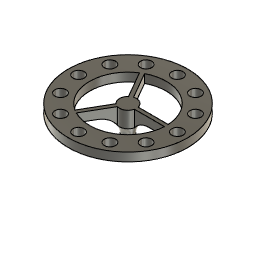
Wheel (Autodesk Fusion 360 design; units mm, degrees)
Autodesk Fusion 360 part; units mm, degrees
sketch "스케치1" plane through (0, 0, 0) normal (0, 0, 1) x (1, 0, 0)
  circle A0 centre (0, 0) radius 1.25
  circle A1 centre (0, 0) radius 3.3
  dimension "d1" = 2.5
  dimension "d2" = 6.6
  constraint coincident A0.centre A1.centre
  measures "d1" diameter of A0
  measures "d2" diameter of A1
extrude "돌출1" add sketch "스케치1" along normal blind 20
sketch "스케치2" plane through (0, 0, 20) normal (0, 0, 1) x (-1, 0, 0)
  circle A0 centre (0, 0) radius 35
  circle A1 centre (0, 0) radius 22.5
  circle A2 centre (0, 0) radius 3.3
  line L0 (-3.0194, -1.0904) -> (-22.4736, -1.0904)
  line L1 (-3.0232, 1.0832) -> (-22.4739, 1.0832)
  circle A3 centre (0, 0) radius 5
  line L2 (2.454, -2.0697) -> (12.1811, -18.9175)
  line L3 (0.5736, -3.1598) -> (10.2989, -20.0046)
  line L4 (0.5654, 3.16) -> (10.2925, 20.0079)
  line L5 (2.4497, 2.0766) -> (12.175, 18.9214)
  dimension "d5" = 70
  dimension "d11" = 45
  dimension "d21" = 10
  dimension "d32" = 360
  constraint coincident A0.centre A1.centre
  constraint concentric A1 A3
  constraint coincident A1 L1.end
  constraint horizontal L1
  constraint coincident A1 L0.end
  constraint horizontal L0
  measures "d5" diameter of A0
  measures "d11" diameter of A1
  measures "d21" diameter of A3
extrude "돌출3" add sketch "스케치2" along normal blind 5 contours A0 | A1 A3 L4 L5 | A1 A3 L2 L3 | A2 A3 L4 L5 | A2 A3 L2 L5 | A2 A3 L2 L3 | A1 L0 L1 A3 | A2 L1 A3 L4 | A2 | A2 L0 A3 L3 | A2 L0 L1 A3
sketch "스케치3" plane through (0, 0, 25) normal (0, 0, 1) x (-1, 0, 0)
  circle A0 centre (-29, 0) radius 3.3
  circle A1 centre (-25.1147, -14.5) radius 3.3
  circle A2 centre (-14.5, -25.1147) radius 3.3
  circle A3 centre (0, -29) radius 3.3
  circle A4 centre (14.5, -25.1147) radius 3.3
  circle A5 centre (25.1147, -14.5) radius 3.3
  circle A6 centre (29, 0) radius 3.3
  circle A7 centre (25.1147, 14.5) radius 3.3
  circle A8 centre (14.5, 25.1147) radius 3.3
  circle A9 centre (0, 29) radius 3.3
  circle A10 centre (-14.5, 25.1147) radius 3.3
  circle A11 centre (-25.1147, 14.5) radius 3.3
  dimension "d33" = 6.6
  dimension "d40" = 360
  measures "d33" diameter of A0
extrude "돌출7" cut sketch "스케치3" against normal through all
fillet "모깎기2" radius 10 1 edges at (-3.0767, -1.1933, 20)
